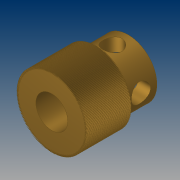
# Autodesk Inventor part: Fillament hob
Saved by Autodesk Inventor 2019 (Build 230136000, 136)
## iProperties
Created: 2018-11-16
Part Number: Fillament hob
Material: Brass, Soft Yellow
Document SubType Name: Modeling
Designer: LillaHunden
Density: 8.47 g/cm^3
Appearance: Brass - Satin
Author: LillaHunden
Autodesk Inventor part; units mm, degrees
ref_plane "XY Plane" through (0, 0, 0) normal (0, 0, 1) x (1, 0, 0)
sketch "Sketch1" plane through (0, 0, 0) normal (0, 0, 1) x (1, 0, 0)
  point P0 (0, 0)
sketch "Sketch2" plane through (0, 0, 0) normal (0, 0, 1) x (1, 0, 0)
  circle A0 centre (0, 0) radius 4.5
  dimension "d0" = 9
  constraints: 1 centre point, 1 coincident
  measures "d0" diameter of A0
extrude "Extrusion1" add sketch "Sketch2" along normal blind 5
sketch "Sketch3" plane through (0, 0, 5) normal (0, 0, 1) x (1, 0, 0)
  circle A0 centre (0, 0) radius 5.5
  dimension "d3" = 11
  constraints: 1 centre point, 1 coincident
  measures "d3" diameter of A0
extrude "Extrusion2" add sketch "Sketch3" along normal blind 7
sketch "Sketch4" plane through (0, 0, 12) normal (0, 0, 1) x (1, 0, 0)
  circle A0 centre (0, 0) radius 5.5 projected
  line L0 (-0.1203, 5.4987) -> (-0.0402, 5.1999)
  line L1 (-0.0402, 5.1999) -> (0.0402, 5.4999)
  arc A1 (0.0402, 5.4999) -> (-0.1203, 5.4987) centre (0, 0) ccw
  circle A2 centre (0, 0) radius 5.5 projected
  line L2 (-0.0402, 5.4999) -> (-0.0402, 5.439)
  dimension "d6" = 0.3
  dimension "d7" = 30
  dimension "d8" = 0.3
  constraints: 6 end point, 5 point on circle, 1 centre point, 1 concentric, 1 vertical, 1 other
  measures "d6" vertical distance of L1.end L0.end
  measures "d7" angle of L0 L1
  measures "d8" distance of L2.start L0.end
extrude "Extrusion3" cut sketch "Sketch4" against normal through all contours L1 L0 A0 picked at (0.0045, 5.3999)
pattern_circular "Circular Pattern1" count 200 over 360 about axis through (0, 0, 0) along (0, 0, 1) of "Extrusion3"
sketch "Sketch5" plane through (0, 0, 12) normal (0, 0, 1) x (1, 0, 0)
  circle A0 centre (0, 0) radius 2.5
  dimension "d14" = 5
  constraints: 1 centre point, 1 coincident
  measures "d14" diameter of A0
extrude "Extrusion4" cut sketch "Sketch5" against normal through all
ref_plane "Work Plane1" through (-4.5, 0, 0) normal (1, 0, 0) x (0, 1, 0)
sketch "Sketch6" plane through (-4.5, 0, 0) normal (1, 0, 0) x (0, 1, 0)
  circle A0 centre (0, 2.5) radius 1.5
  line L0 (0, 0) -> (0, 5)
  line L1 (4.5, 5) -> (-4.5, 5) projected
  point P0 (0, 2.5)
  dimension "d17" = 3
  constraints: 2 end point, 2 midpoint, 1 centre point, 1 coincident
  measures "d17" diameter of A0
extrude "Extrusion5" cut sketch "Sketch6" along normal through all
ref_plane "Work Plane2" through (0, 4.5, 0) normal (0, 1, 0) x (-1, 0, 0)
sketch "Sketch7" plane through (0, 4.5, 0) normal (0, 1, 0) x (-1, 0, 0)
  line L0 (0.0402, 5) -> (-0.0402, 5) projected
  line L1 (0, 5) -> (0, 0)
  circle A0 centre (0, 2.5) radius 1.5
  point P0 (0, 2.5)
  dimension "d20" = 3
  constraints: 3 midpoint, 2 end point, 1 centre point, 1 coincident, 1 vertical
  measures "d20" diameter of A0
extrude "Extrusion6" cut sketch "Sketch7" against normal blind 4.5
body "Solid1"
